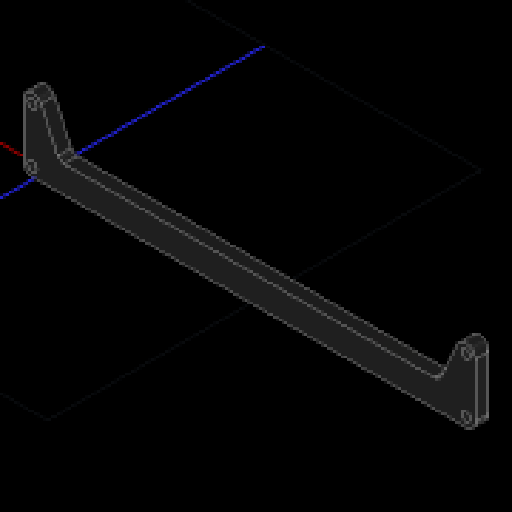
# Autodesk Inventor part: brace
Saved by Autodesk Inventor 2025.2 (Build 292293000, 293)
## iProperties
Created: 2026-01-12
Part Number: brace
Material: Acetal Resin, Black
Document SubType Name: Modeling
Designer: cloudy
Density: 1.425 g/cm^3
Appearance: Smooth - Black
Author: cloudy
Autodesk Inventor part; units mm, degrees
ref_plane "YZ Plane" through (0, 0, 0) normal (1, 0, 0) x (0, 1, 0)
ref_plane "XZ Plane" through (0, 0, 0) normal (0, 1, 0) x (-1, 0, 0)
ref_plane "XY Plane" through (0, 0, 0) normal (0, 0, 1) x (1, 0, 0)
sketch "Sketch1" plane through (0, 0, 0) normal (0, 0, 1) x (1, 0, 0)
  circle A0 centre (-0.7751, 114.3) radius 2.1844 projected
  circle A1 centre (-0.7751, 139.7) radius 2.1844 projected
  circle A2 centre (202.4249, 139.7) radius 2.1844 projected
  circle A3 centre (202.4249, 114.3) radius 2.1844 projected
  arc A4 (-5.2201, 114.3) -> (-0.7751, 109.855) centre (-0.7751, 114.3) ccw
  circle A5 centre (-0.7751, 139.7) radius 4.445
  arc A6 (206.8699, 139.7) -> (198.7471, 142.1965) centre (202.4249, 139.7) ccw
  arc A7 (202.4249, 109.855) -> (206.8699, 114.3) centre (202.4249, 114.3) ccw
  line L0 (202.4249, 109.855) -> (-0.7751, 109.855)
  line L1 (-5.2201, 114.3) -> (-5.2201, 139.7)
  line L2 (2.9026, 142.1965) -> (10.9801, 130.2968)
  line L3 (13.607, 128.905) -> (188.0427, 128.905)
  line L4 (190.6696, 130.2968) -> (198.7471, 142.1965)
  line L5 (206.8699, 140.9911) -> (206.8699, 114.3)
  arc A8 (188.0427, 128.905) -> (190.6696, 130.2968) centre (188.0427, 132.08) ccw
  arc A9 (10.9801, 130.2968) -> (13.607, 128.905) centre (13.607, 132.08) ccw
  point P0 (0, 0)
  point P1 (11.9249, 128.905)
  point P2 (189.7249, 128.905)
  dimension "d0" = 8.89
  dimension "d2" = 19.05
  dimension "d3" = 177.8
  dimension "d4" = 3.175
  constraints: 12 end point, 12 point on circle, 10 tangent, 6 centre point, 5 point on line, 4 coincident, 4 equal radius, 2 vertical, 1 equal length, 1 parallel
  measures "d0" diameter of A4
  measures "d2" distance between parallel lines of L0 L3
  measures "d3" distance of point (11.925, 128.905) point (189.725, 128.905)
  measures "d4" radius of A8
extrude "Extrusion1" add sketch "Sketch1" along normal blind 6.35
body "Solid1"
